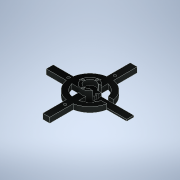
# Autodesk Inventor part: prindere senzor
Saved by Autodesk Inventor 2022 (Build 260153000, 153)
## iProperties
Created: 2022-02-27
Part Number: prindere senzor
Material: Generic
Document SubType Name: Modeling
Designer: Oana
Density: 1 g/cm^3
Appearance: Gunmetal - Polished
Author: Oana
Autodesk Inventor part; units mm, degrees
ref_plane "YZ Plane" through (0, 0, 0) normal (1, 0, 0) x (0, 1, 0)
ref_plane "XZ Plane" through (0, 0, 0) normal (0, 1, 0) x (-1, 0, 0)
ref_plane "XY Plane" through (0, 0, 0) normal (0, 0, 1) x (1, 0, 0)
sketch "Sketch1" plane through (0, 0, 0) normal (0, 1, 0) x (-1, 0, 0)
  circle A0 centre (0, 0) radius 9.5
  line L0 (-3.8533, 8.6834) -> (-3.8533, 38.6834)
  line L1 (-7.8533, -5.3457) -> (-7.8533, 38.6834)
  line L2 (-7.8533, 38.6834) -> (-3.8533, 38.6834)
  line L3 (-5.8533, 7.4826) -> (-5.8533, 50.3065) construction
  line L4 (-3.8533, 38.6834) -> (-7.8533, -5.3457) construction
  line L5 (-7.8533, 38.6834) -> (-3.8533, 8.6834) construction
  line L6 (-2.7738, -9.086) -> (-2.7738, -39.086)
  line L7 (-2.7738, -39.086) -> (-6.7738, -39.086)
  line L8 (-6.7738, -39.086) -> (-6.7738, 6.6608)
  point P0 (-5.8533, 16.6689)
  dimension "d0" = 19
  dimension "d10" = 30
  dimension "d16" = 4
  constraints: 18 end point, 5 point on circle, 3 perpendicular, 3 vertical, 2 parallel, 1 centre point, 1 coincident, 1 horizontal, 1 midpoint, 1 point on line
  measures "d0" diameter of A0
  measures "d10" distance of L0.start L0.end
  measures "d16" distance of L1.end L0.end
extrude "Extrusion1" add sketch "Sketch1" along normal blind 3 contours A0 L8 | L8 A0 L1 | L1 A0
sketch "Sketch2" plane through (0, 3, 0) normal (0, 1, 0) x (1, 0, 0)
  circle A0 centre (0, 0) radius 6.5
  circle A1 centre (0, 0) radius 9.5 projected
  dimension "d3" = 3
  constraints: 1 centre point, 1 coincident
  measures "d3" radial gap between concentric circles of A1 A0
extrude "Extrusion2" add sketch "Sketch2" along normal blind 4
sketch "Sketch3" plane through (0, 7, 0) normal (0, 1, 0) x (1, 0, 0)
  line L0 (4.6242, -5) -> (32.9242, -5)
  line L1 (32.9242, -5) -> (32.9242, 5)
  line L2 (32.9242, 5) -> (4.6242, 5)
  line L3 (4.6242, 5) -> (4.6242, -5)
  line L4 (4.6242, -5) -> (32.9242, 5)
  line L5 (4.6242, 5) -> (32.9242, -5)
  line L6 (0, 0) -> (18.7742, 0)
  dimension "d6" = 10
  dimension "d7" = 28.3
  constraints: 14 end point, 2 horizontal, 2 parallel, 1 coincident, 1 midpoint, 1 perpendicular
  measures "d6" distance of L2.end L0.start
  measures "d7" distance of L1.end L2.end
extrude "Extrusion3" cut sketch "Sketch3" against normal blind 5
sketch "Sketch5" plane through (0, 0, 0) normal (0, -1, 0) x (1, 0, 0)
  line L0 (0, 42.0095) -> (0, -66.9743)
  line L1 (-60.4099, 0) -> (61.9955, 0)
  line L2 (-4, 50) -> (4, 50)
  line L3 (4, 50) -> (4, 0)
  line L4 (4, 0) -> (-4, 0)
  line L5 (-4, 0) -> (-4, 50)
  line L6 (-4, 50) -> (4, 0) construction
  line L7 (4, 50) -> (-4, 0) construction
  line L8 (4, -50) -> (-4, -50)
  line L9 (-4, -50) -> (-4, 0)
  line L10 (-4, 0) -> (4, 0)
  line L11 (4, 0) -> (4, -50)
  line L12 (4, -50) -> (-4, 0) construction
  line L13 (-4, -50) -> (4, 0) construction
  line L14 (-46, 4) -> (-4, 4)
  line L15 (-4, 4) -> (-4, -4)
  line L16 (-4, -4) -> (-46, -4)
  line L17 (-46, -4) -> (-46, 4)
  line L18 (-46, 4) -> (-4, -4) construction
  line L19 (-4, 4) -> (-46, -4) construction
  line L20 (46, 4) -> (4, 4)
  line L21 (4, 4) -> (4, -4)
  line L22 (4, -4) -> (46, -4)
  line L23 (46, -4) -> (46, 4)
  line L24 (46, 4) -> (4, -4) construction
  line L25 (4, 4) -> (46, -4) construction
  point P0 (0, 0)
  point P1 (0, 25)
  point P2 (0, -25)
  point P3 (-25, 0)
  point P4 (25, 0)
  point P5 (4, 4)
  point P6 (-4, 4)
  dimension "d17" = 8
  dimension "d18" = 50
  dimension "d19" = 50
  dimension "d20" = 8
  dimension "d21" = 42
  dimension "d22" = 42
  dimension "d23" = 8
  constraints: 52 end point, 8 midpoint, 8 parallel, 8 point on line, 6 horizontal, 4 perpendicular, 1 vertical
  measures "d17" distance between parallel lines of L3 L5
  measures "d18" distance of L2.end L3.end
  measures "d19" distance of L10.end L8.start
  measures "d20" distance of L16.end L14.start
  measures "d21" distance of L14.start L14.end
  measures "d22" distance of L20.start L20.end
  measures "d23" distance of L22.end L20.start
extrude "Extrusion5" add sketch "Sketch5" against normal blind 6
sketch "Sketch6" plane through (0, 6, 0) normal (0, 1, 0) x (1, 0, 0)
  line L0 (8.6568, 5.0074) -> (46.1585, 5.0074)
  line L1 (46.1585, 5.0074) -> (46.1585, -5.1816)
  line L2 (46.1585, -5.1816) -> (8.6568, -5.1816)
  line L3 (8.6568, -5.1816) -> (8.6568, 5.0074)
  point P0 (0, 0)
  constraints: 8 end point, 2 parallel, 1 horizontal, 1 perpendicular
extrude "Extrusion6" cut sketch "Sketch6" against normal blind 4
sketch "Sketch7" plane through (0, 0, 0) normal (0, -1, 0) x (1, 0, 0)
  circle A0 centre (-8, 0) radius 1.35 projected
  circle A1 centre (0, 8) radius 1.35 projected
  circle A2 centre (8, 0) radius 1.35 projected
  arc A3 (-8.6168, -4) -> (-4, -8.6168) centre (0, 0) ccw projected
  line L0 (-4, -8.6168) -> (-4, -50) projected
  line L1 (-4, -50) -> (4, -50) projected
  line L2 (4, -50) -> (4, -8.6168) projected
  arc A4 (4, -8.6168) -> (8.6168, -4) centre (0, 0) ccw projected
  line L3 (8.6168, -4) -> (46, -4) projected
  line L4 (46, -4) -> (46, 4) projected
  line L5 (46, 4) -> (8.6168, 4) projected
  arc A5 (8.6168, 4) -> (4, 8.6168) centre (0, 0) ccw projected
  line L6 (4, 8.6168) -> (4, 50) projected
  line L7 (4, 50) -> (-4, 50) projected
  line L8 (-4, 50) -> (-4, 8.6168) projected
  arc A6 (-4, 8.6168) -> (-8.6168, 4) centre (0, 0) ccw projected
  line L9 (-8.6168, 4) -> (-46, 4) projected
  line L10 (-46, 4) -> (-46, -4) projected
  line L11 (-46, -4) -> (-8.6168, -4) projected
  circle A7 centre (0, -8) radius 1.35 projected
extrude "Extrusion7" cut sketch "Sketch7" against normal through all contours A0 | A1 | A2 | A7
sketch "Sketch8" plane through (0, 0, 0) normal (0, -1, 0) x (1, 0, 0)
  circle A0 centre (0, 28.5) radius 1.5
  line L0 (4, 50) -> (-4, 50) projected
  circle A1 centre (-24.5, 0) radius 1.5
  circle A2 centre (24.5, 0) radius 1.5
  line L1 (0, 50) -> (0, 30)
  line L2 (-46, 0) -> (-26, 0)
  line L3 (-46, 4) -> (-46, -4) projected
  line L4 (26, 0) -> (46, 0)
  line L5 (46, -4) -> (46, 4) projected
  circle A3 centre (0, -28.5) radius 1.5
  line L6 (0, -30) -> (0, -50)
  line L7 (-4, -50) -> (4, -50) projected
  point P0 (0, 0)
  dimension "d30" = 3
  dimension "d32" = 20
  constraints: 8 end point, 4 midpoint, 3 perpendicular, 2 horizontal, 2 horizontal alignment, 2 vertical, 2 vertical alignment, 8 other
  measures "d32" distance of L1.start L1.end
extrude "Extrusion8" cut sketch "Sketch8" against normal through all contours A0 | A1 | A3
sketch "Sketch9" plane through (0, 7, 0) normal (0, 1, 0) x (1, 0, 0)
  circle A0 centre (0, -8) radius 1.35 projected
  circle A1 centre (-8, 0) radius 1.35 projected
  circle A2 centre (0, 8) radius 1.35 projected
  line L0 (8.0777, -5) -> (4.6242, -5) projected
  line L1 (4.6242, -5) -> (4.6242, -4.5681) projected
  arc A3 (4.6242, 4.5681) -> (4.6242, -4.5681) centre (0, 0) ccw projected
  line L2 (4.6242, 4.5681) -> (4.6242, 5) projected
  line L3 (4.6242, 5) -> (8.0777, 5) projected
  arc A4 (8.0777, 5) -> (8.0777, -5) centre (0, 0) ccw projected
extrude "Extrusion9" add sketch "Sketch9" along normal blind 5
sketch "Sketch10" plane through (0, 0, 0) normal (0, -1, 0) x (1, 0, 0)
  circle A0 centre (0, 0) radius 23.4467
  circle A1 centre (0, 0) radius 17.1503
  constraints: 2 centre point, 2 coincident
extrude "Extrusion10" add sketch "Sketch10" against normal up to surface (6 mm away)
sketch "Sketch11" plane through (0, 6, 0) normal (0, 1, 0) x (1, 0, 0)
  arc A0 (23.103, -4) -> (23.103, 4) centre (0, 0) ccw projected
  line L0 (46, -4) -> (23.103, -4) projected
  line L1 (46, 4) -> (46, -4) projected
  line L2 (23.103, 4) -> (46, 4) projected
  arc A1 (16.6773, -4) -> (16.6773, 4) centre (0, 0) ccw projected
  line L3 (8.6568, 4) -> (16.6773, 4) projected
  line L4 (8.6568, 1.1794) -> (8.6568, 4) projected
  arc A2 (8.6568, -1.1794) -> (8.6568, 1.1794) centre (8, 0) ccw projected
  line L5 (8.6568, -4) -> (8.6568, -1.1794) projected
  line L6 (16.6773, -4) -> (8.6568, -4) projected
  line L7 (23.103, 4) -> (16.6773, 4)
  line L8 (23.103, -4) -> (16.6773, -4)
  arc A3 (23.103, -4) -> (23.103, 4) centre (0, 0) ccw
  arc A4 (16.6773, -4) -> (16.6773, 4) centre (0, 0) ccw
  constraints: 4 end point, 4 point on circle, 2 centre point, 2 collinear, 2 concentric
extrude "Extrusion11" cut sketch "Sketch11" against normal up to surface (4 mm away) contours L8 A1 L7 A0
body "Solid1"
